Autodesk Inventor part; units mm, degrees
(part 2 of 2)
sketch "Sketch10" plane through (0, 0, 0) normal (1, 0, 0) x (0, 0, -1)
  line L0 (200.5868, 90.5719) -> (65.5868, 90.5719) projected
  arc A0 (65.5868, 90.5719) -> (50.5868, 90.5719) centre (58.0868, 90.5719) ccw projected
  line L1 (50.5868, 90.5719) -> (-146.9132, 90.5719) projected
  arc A1 (-146.9132, 90.5719) -> (-164.5909, 47.8942) centre (-146.9132, 65.5719) ccw projected
  line L2 (-164.5909, 47.8942) -> (-120.1975, 3.5008) projected
  arc A2 (-120.1975, 3.5008) -> (-113.1264, 0.5719) centre (-113.1264, 10.5719) ccw projected
  line L3 (-113.1264, 0.5719) -> (48.2351, 0.5719) projected
  arc A3 (48.2351, 0.5719) -> (67.9385, 0.5719) centre (58.0868, 2.2876) ccw projected
  line L4 (67.9385, 0.5719) -> (198.2351, 0.5719) projected
  arc A4 (198.2351, 0.5719) -> (217.9385, 0.5719) centre (208.0868, 2.2876) ccw projected
  line L5 (217.9385, 0.5719) -> (338.2351, 0.5719) projected
  arc A5 (338.2351, 0.5719) -> (357.9385, 0.5719) centre (348.0868, 2.2876) ccw projected
  line L6 (357.9385, 0.5719) -> (387.824, 0.5719) projected
  arc A6 (387.824, 0.5719) -> (392.824, 1.9116) centre (387.824, 10.5719) ccw projected
  line L7 (392.824, 1.9116) -> (465.5868, 43.9213) projected
  arc A7 (465.5868, 43.9213) -> (453.0868, 90.5719) centre (453.0868, 65.5719) ccw projected
  line L8 (453.0868, 90.5719) -> (215.5868, 90.5719) projected
  arc A8 (215.5868, 90.5719) -> (200.5868, 90.5719) centre (208.0868, 90.5719) ccw projected
  line L9 (394.4234, 30.0809) -> (384.8369, 44.4607) projected
  arc A9 (384.8369, 46.6796) -> (384.8369, 44.4607) centre (386.501, 45.5701) ccw projected
  line L10 (384.8369, 46.6796) -> (394.4264, 61.0622) projected
  arc A10 (398.0904, 59.9525) -> (394.4264, 61.0622) centre (396.0904, 59.9527) ccw projected
  line L11 (398.0904, 59.9525) -> (398.0875, 31.1901) projected
  arc A11 (394.4234, 30.0809) -> (398.0875, 31.1901) centre (396.0875, 31.1903) ccw projected
  line L12 (-95.7021, 34.3299) -> (-100.8758, 44.6775) projected
  arc A12 (-100.8758, 46.4663) -> (-100.8758, 44.6775) centre (-99.087, 45.5719) ccw projected
  line L13 (-100.8758, 46.4663) -> (-95.7021, 56.8138) projected
  arc A13 (-91.9132, 55.9194) -> (-95.7021, 56.8138) centre (-93.9132, 55.9194) ccw projected
  line L14 (-91.9132, 55.9194) -> (-91.9132, 35.2244) projected
  arc A14 (-95.7021, 34.3299) -> (-91.9132, 35.2244) centre (-93.9132, 35.2244) ccw projected
  line L15 (46.0868, 47.6815) -> (11.9586, 47.6815) projected
  arc A15 (11.0641, 51.4704) -> (11.9586, 47.6815) centre (11.9586, 49.6815) ccw projected
  line L16 (11.0641, 51.4704) -> (45.1924, 68.5345) projected
  arc A16 (48.0868, 66.7457) -> (45.1924, 68.5345) centre (46.0868, 66.7457) ccw projected
  line L17 (48.0868, 66.7457) -> (48.0868, 49.6815) projected
  arc A17 (46.0868, 47.6815) -> (48.0868, 49.6815) centre (46.0868, 49.6815) ccw projected
  line L18 (278.9812, 39.5345) -> (319.3287, 19.3608) projected
  arc A18 (318.4343, 15.5719) -> (319.3287, 19.3608) centre (318.4343, 17.5719) ccw projected
  line L19 (318.4343, 15.5719) -> (237.7393, 15.5719) projected
  arc A19 (236.8448, 19.3608) -> (237.7393, 15.5719) centre (237.7393, 17.5719) ccw projected
  line L20 (236.8448, 19.3608) -> (277.1924, 39.5345) projected
  arc A20 (278.9812, 39.5345) -> (277.1924, 39.5345) centre (278.0868, 37.7457) ccw projected
  line L21 (367.8331, 75.5719) -> (388.3444, 75.5719) projected
  arc A21 (390.0084, 72.4624) -> (388.3444, 75.5719) centre (388.3444, 73.5719) ccw projected
  line L22 (390.0084, 72.4624) -> (379.7522, 57.0798) projected
  arc A22 (376.4241, 57.0798) -> (379.7522, 57.0798) centre (378.0882, 58.1892) ccw projected
  line L23 (376.4241, 57.0798) -> (366.169, 72.4625) projected
  arc A23 (367.8331, 75.5719) -> (366.169, 72.4625) centre (367.8331, 73.5719) ccw projected
  line L24 (361.7509, 61.0619) -> (371.3389, 46.6799) projected
  arc A24 (371.3388, 44.461) -> (371.3389, 46.6799) centre (369.6748, 45.5705) ccw projected
  line L25 (371.3388, 44.461) -> (361.7508, 30.0806) projected
  arc A25 (358.0868, 31.1901) -> (361.7508, 30.0806) centre (360.0868, 31.1901) ccw projected
  line L26 (358.0868, 31.1901) -> (358.0868, 59.9525) projected
  arc A26 (361.7509, 61.0619) -> (358.0868, 59.9525) centre (360.0868, 59.9525) ccw projected
  line L27 (89.1243, 75.5719) -> (177.0493, 75.5719) projected
  arc A27 (177.8875, 71.756) -> (177.0493, 75.5719) centre (177.0493, 73.5719) ccw projected
  line L28 (177.8875, 71.756) -> (133.9249, 51.4656) projected
  arc A28 (132.2487, 51.4656) -> (133.9249, 51.4656) centre (133.0868, 53.2815) ccw projected
  line L29 (132.2487, 51.4656) -> (88.2861, 71.756) projected
  arc A29 (89.1243, 75.5719) -> (88.2861, 71.756) centre (89.1243, 73.5719) ccw projected
  line L30 (-11.0188, 39.5345) -> (29.3287, 19.3608) projected
  arc A30 (28.4343, 15.5719) -> (29.3287, 19.3608) centre (28.4343, 17.5719) ccw projected
  line L31 (28.4343, 15.5719) -> (-52.2607, 15.5719) projected
  arc A31 (-53.1552, 19.3608) -> (-52.2607, 15.5719) centre (-52.2607, 17.5719) ccw projected
  line L32 (-53.1552, 19.3608) -> (-12.8076, 39.5345) projected
  arc A32 (-11.0188, 39.5345) -> (-12.8076, 39.5345) centre (-11.9132, 37.7457) ccw projected
  line L33 (-105.1244, 30.8138) -> (-98.9506, 18.4663) projected
  arc A33 (-100.7394, 15.5719) -> (-98.9506, 18.4663) centre (-100.7394, 17.5719) ccw projected
  line L34 (-100.7394, 15.5719) -> (-113.087, 15.5719) projected
  arc A34 (-114.8758, 18.4663) -> (-113.087, 15.5719) centre (-113.087, 17.5719) ccw projected
  line L35 (-114.8758, 18.4663) -> (-108.7021, 30.8138) projected
  arc A35 (-105.1244, 30.8138) -> (-108.7021, 30.8138) centre (-106.9132, 29.9194) ccw projected
  line L36 (117.2208, 43.756) -> (70.9249, 22.3887) projected
  arc A36 (68.0868, 24.2046) -> (70.9249, 22.3887) centre (70.0868, 24.2046) ccw projected
  line L37 (68.0868, 24.2046) -> (68.0868, 66.9392) projected
  arc A37 (70.9249, 68.7551) -> (68.0868, 66.9392) centre (70.0868, 66.9392) ccw projected
  line L38 (70.9249, 68.7551) -> (117.2208, 47.3878) projected
  arc A38 (117.2208, 43.756) -> (117.2208, 47.3878) centre (116.3827, 45.5719) ccw projected
  line L39 (-118.1244, 56.8138) -> (-112.9506, 46.4663) projected
  arc A39 (-112.9506, 44.6775) -> (-112.9506, 46.4663) centre (-114.7394, 45.5719) ccw projected
  line L40 (-112.9506, 44.6775) -> (-118.1244, 34.3299) projected
  arc A40 (-121.9132, 35.2244) -> (-118.1244, 34.3299) centre (-119.9132, 35.2244) ccw projected
  line L41 (-121.9132, 35.2244) -> (-121.9132, 55.9194) projected
  arc A41 (-118.1244, 56.8138) -> (-121.9132, 55.9194) centre (-119.9132, 55.9194) ccw projected
  line L42 (-71.9132, 24.3981) -> (-71.9132, 66.7457) projected
  arc A42 (-69.0188, 68.5345) -> (-71.9132, 66.7457) centre (-69.9132, 66.7457) ccw projected
  line L43 (-69.0188, 68.5345) -> (-26.6713, 47.3608) projected
  arc A43 (-26.6713, 43.783) -> (-26.6713, 47.3608) centre (-27.5657, 45.5719) ccw projected
  line L44 (-26.6713, 43.783) -> (-69.0188, 22.6093) projected
  arc A44 (-71.9132, 24.3981) -> (-69.0188, 22.6093) centre (-69.9132, 24.3981) ccw projected
  line L45 (177.0493, 15.5719) -> (89.1243, 15.5719) projected
  arc A45 (88.2861, 19.3878) -> (89.1243, 15.5719) centre (89.1243, 17.5719) ccw projected
  line L46 (88.2861, 19.3878) -> (132.2487, 39.6782) projected
  arc A46 (133.9249, 39.6782) -> (132.2487, 39.6782) centre (133.0868, 37.8623) ccw projected
  line L47 (133.9249, 39.6782) -> (177.8875, 19.3878) projected
  arc A47 (177.0493, 15.5719) -> (177.8875, 19.3878) centre (177.0493, 17.5719) ccw projected
  line L48 (330.1924, 25.1093) -> (292.8448, 43.783) projected
  arc A48 (292.8448, 47.3608) -> (292.8448, 43.783) centre (293.7393, 45.5719) ccw projected
  line L49 (292.8448, 47.3608) -> (330.1924, 66.0345) projected
  arc A49 (333.0868, 64.2457) -> (330.1924, 66.0345) centre (331.0868, 64.2457) ccw projected
  line L50 (333.0868, 64.2457) -> (333.0868, 26.8981) projected
  arc A50 (330.1924, 25.1093) -> (333.0868, 26.8981) centre (331.0868, 26.8981) ccw projected
  line L51 (379.7517, 34.0607) -> (390.0046, 18.6813) projected
  arc A51 (388.3405, 15.5719) -> (390.0046, 18.6813) centre (388.3405, 17.5719) ccw projected
  line L52 (388.3405, 15.5719) -> (367.8335, 15.5719) projected
  arc A52 (366.1695, 18.6814) -> (367.8335, 15.5719) centre (367.8335, 17.5719) ccw projected
  line L53 (366.1695, 18.6814) -> (376.4235, 34.0608) projected
  arc A53 (379.7517, 34.0607) -> (376.4235, 34.0608) centre (378.0876, 32.9513) ccw projected
  line L54 (237.7393, 75.5719) -> (318.4343, 75.5719) projected
  arc A54 (319.3287, 71.783) -> (318.4343, 75.5719) centre (318.4343, 73.5719) ccw projected
  line L55 (319.3287, 71.783) -> (278.9812, 51.6093) projected
  arc A55 (277.1924, 51.6093) -> (278.9812, 51.6093) centre (278.0868, 53.3981) ccw projected
  line L56 (277.1924, 51.6093) -> (236.8448, 71.783) projected
  arc A56 (237.7393, 75.5719) -> (236.8448, 71.783) centre (237.7393, 73.5719) ccw projected
  line L57 (196.0868, 47.6815) -> (158.6952, 47.6815) projected
  arc A57 (157.857, 51.4975) -> (158.6952, 47.6815) centre (158.6952, 49.6815) ccw projected
  line L58 (157.857, 51.4975) -> (195.2487, 68.7551) projected
  arc A58 (198.0868, 66.9392) -> (195.2487, 68.7551) centre (196.0868, 66.9392) ccw projected
  line L59 (198.0868, 66.9392) -> (198.0868, 49.6815) projected
  arc A59 (196.0868, 47.6815) -> (198.0868, 49.6815) centre (196.0868, 49.6815) ccw projected
  line L60 (-52.2607, 75.5719) -> (28.4343, 75.5719) projected
  arc A60 (29.3287, 71.783) -> (28.4343, 75.5719) centre (28.4343, 73.5719) ccw projected
  line L61 (29.3287, 71.783) -> (-11.0188, 51.6093) projected
  arc A61 (-12.8076, 51.6093) -> (-11.0188, 51.6093) centre (-11.9132, 53.3981) ccw projected
  line L62 (-12.8076, 51.6093) -> (-53.1552, 71.783) projected
  arc A62 (-52.2607, 75.5719) -> (-53.1552, 71.783) centre (-52.2607, 73.5719) ccw projected
  line L63 (-98.9506, 72.6775) -> (-105.1244, 60.3299) projected
  arc A63 (-108.7021, 60.3299) -> (-105.1244, 60.3299) centre (-106.9132, 61.2244) ccw projected
  line L64 (-108.7021, 60.3299) -> (-114.8758, 72.6775) projected
  arc A64 (-113.087, 75.5719) -> (-114.8758, 72.6775) centre (-113.087, 73.5719) ccw projected
  line L65 (-113.087, 75.5719) -> (-100.7394, 75.5719) projected
  arc A65 (-98.9506, 72.6775) -> (-100.7394, 75.5719) centre (-100.7394, 73.5719) ccw projected
  line L66 (220.9812, 68.5345) -> (263.3287, 47.3608) projected
  arc A66 (263.3287, 43.783) -> (263.3287, 47.3608) centre (262.4343, 45.5719) ccw projected
  line L67 (263.3287, 43.783) -> (220.9812, 22.6093) projected
  arc A67 (218.0868, 24.3981) -> (220.9812, 22.6093) centre (220.0868, 24.3981) ccw projected
  line L68 (218.0868, 24.3981) -> (218.0868, 66.7457) projected
  arc A68 (220.9812, 68.5345) -> (218.0868, 66.7457) centre (220.0868, 66.7457) ccw projected
  circle A69 centre (208.0868, 2.2876) radius 2.5 projected
  circle A70 centre (348.0868, 2.2876) radius 2.5 projected
  circle A71 centre (243.0868, 8.0719) radius 2.5 projected
  circle A72 centre (183.0868, 37.6815) radius 2.5 projected
  circle A73 centre (23.0868, 37.6815) radius 2.5 projected
  circle A74 centre (-81.9132, 83.0719) radius 2.5 projected
  circle A75 centre (-122.4179, 16.3278) radius 2.5 projected
  circle A76 centre (100.0868, 83.0715) radius 2.5 projected
  circle A77 centre (260.0868, 83.0715) radius 2.5 projected
  circle A78 centre (343.0868, 37.6815) radius 2.5 projected
  circle A79 centre (348.0868, 83.0719) radius 2.5 projected
  circle A80 centre (58.0868, 2.2876) radius 2.5 projected
  circle A81 centre (-81.9132, 8.0719) radius 2.5 projected
  circle A82 centre (-146.9132, 65.5719) radius 11 projected
  line L69 (413.0868, 68.5719) -> (453.0868, 68.5719) projected
  arc A83 (453.0868, 62.5719) -> (453.0868, 68.5719) centre (453.0868, 65.5719) ccw projected
  line L70 (453.0868, 62.5719) -> (413.0868, 62.5719) projected
  arc A84 (413.0868, 68.5719) -> (413.0868, 62.5719) centre (413.0868, 65.5719) ccw projected
  line L71 (-71.9132, 24.3981) -> (-71.9132, 66.7457) projected
  line L72 (-71.9132, 24.3981) -> (-91.9132, 24.3981)
  line L73 (-91.9132, 24.3981) -> (-91.9132, 90.5719)
  line L74 (-91.9132, 90.5719) -> (-71.9132, 90.5719)
  line L75 (-71.9132, 90.5719) -> (-71.9132, 24.3981)
  line L76 (-91.9132, 90.5719) -> (-71.9132, 90.5719)
  line L77 (-71.9132, 90.5719) -> (-71.9132, -7.7124)
  line L78 (-71.9132, -7.7124) -> (-91.9132, -7.7124)
  line L79 (-91.9132, -7.7124) -> (-91.9132, 90.5719)
  line L80 (-71.9132, 90.5719) -> (-91.9132, 90.5719)
  line L81 (-91.9132, 90.5719) -> (-91.9132, 103.5219)
  line L82 (-91.9132, 103.5219) -> (-71.9132, 103.5219)
  line L83 (-71.9132, 103.5219) -> (-71.9132, 90.5719)
  point P0 (0, 0)
  point P1 (-91.9132, 0.5719)
  dimension "d165" = 20
  constraints: 24 end point, 6 parallel, 3 horizontal, 3 perpendicular, 3 point on line
  measures "d165" distance of L73.end L74.end
extrude "Extrusion4" cut sketch "Sketch10" against normal blind 10 contours L73 A13 L13 A12 L12 A14 L79 L3 A2 L2 A1 L1
sketch "Sketch11" plane through (0, 0, 0) normal (1, 0, 0) x (0, 0, -1)
  line L0 (-91.9132, 90.5719) -> (-91.9132, 0.5719) projected
  line L1 (-91.9132, 0.5719) -> (48.2351, 0.5719) projected
  arc A0 (48.2351, 0.5719) -> (67.9385, 0.5719) centre (58.0868, 2.2876) ccw projected
  line L2 (67.9385, 0.5719) -> (198.2351, 0.5719) projected
  arc A1 (198.2351, 0.5719) -> (217.9385, 0.5719) centre (208.0868, 2.2876) ccw projected
  line L3 (217.9385, 0.5719) -> (338.2351, 0.5719) projected
  arc A2 (338.2351, 0.5719) -> (357.9385, 0.5719) centre (348.0868, 2.2876) ccw projected
  line L4 (357.9385, 0.5719) -> (387.824, 0.5719) projected
  arc A3 (387.824, 0.5719) -> (392.824, 1.9116) centre (387.824, 10.5719) ccw projected
  line L5 (392.824, 1.9116) -> (465.5868, 43.9213) projected
  arc A4 (465.5868, 43.9213) -> (453.0868, 90.5719) centre (453.0868, 65.5719) ccw projected
  line L6 (453.0868, 90.5719) -> (215.5868, 90.5719) projected
  arc A5 (215.5868, 90.5719) -> (200.5868, 90.5719) centre (208.0868, 90.5719) ccw projected
  line L7 (200.5868, 90.5719) -> (65.5868, 90.5719) projected
  arc A6 (65.5868, 90.5719) -> (50.5868, 90.5719) centre (58.0868, 90.5719) ccw projected
  line L8 (50.5868, 90.5719) -> (-91.9132, 90.5719) projected
  line L9 (394.4234, 30.0809) -> (384.8369, 44.4607) projected
  arc A7 (384.8369, 46.6796) -> (384.8369, 44.4607) centre (386.501, 45.5701) ccw projected
  line L10 (384.8369, 46.6796) -> (394.4264, 61.0622) projected
  arc A8 (398.0904, 59.9525) -> (394.4264, 61.0622) centre (396.0904, 59.9527) ccw projected
  line L11 (398.0904, 59.9525) -> (398.0875, 31.1901) projected
  arc A9 (394.4234, 30.0809) -> (398.0875, 31.1901) centre (396.0875, 31.1903) ccw projected
  line L12 (46.0868, 47.6815) -> (11.9586, 47.6815) projected
  arc A10 (11.0641, 51.4704) -> (11.9586, 47.6815) centre (11.9586, 49.6815) ccw projected
  line L13 (11.0641, 51.4704) -> (45.1924, 68.5345) projected
  arc A11 (48.0868, 66.7457) -> (45.1924, 68.5345) centre (46.0868, 66.7457) ccw projected
  line L14 (48.0868, 66.7457) -> (48.0868, 49.6815) projected
  arc A12 (46.0868, 47.6815) -> (48.0868, 49.6815) centre (46.0868, 49.6815) ccw projected
  line L15 (278.9812, 39.5345) -> (319.3287, 19.3608) projected
  arc A13 (318.4343, 15.5719) -> (319.3287, 19.3608) centre (318.4343, 17.5719) ccw projected
  line L16 (318.4343, 15.5719) -> (237.7393, 15.5719) projected
  arc A14 (236.8448, 19.3608) -> (237.7393, 15.5719) centre (237.7393, 17.5719) ccw projected
  line L17 (236.8448, 19.3608) -> (277.1924, 39.5345) projected
  arc A15 (278.9812, 39.5345) -> (277.1924, 39.5345) centre (278.0868, 37.7457) ccw projected
  line L18 (367.8331, 75.5719) -> (388.3444, 75.5719) projected
  arc A16 (390.0084, 72.4624) -> (388.3444, 75.5719) centre (388.3444, 73.5719) ccw projected
  line L19 (390.0084, 72.4624) -> (379.7522, 57.0798) projected
  arc A17 (376.4241, 57.0798) -> (379.7522, 57.0798) centre (378.0882, 58.1892) ccw projected
  line L20 (376.4241, 57.0798) -> (366.169, 72.4625) projected
  arc A18 (367.8331, 75.5719) -> (366.169, 72.4625) centre (367.8331, 73.5719) ccw projected
  line L21 (361.7509, 61.0619) -> (371.3389, 46.6799) projected
  arc A19 (371.3388, 44.461) -> (371.3389, 46.6799) centre (369.6748, 45.5705) ccw projected
  line L22 (371.3388, 44.461) -> (361.7508, 30.0806) projected
  arc A20 (358.0868, 31.1901) -> (361.7508, 30.0806) centre (360.0868, 31.1901) ccw projected
  line L23 (358.0868, 31.1901) -> (358.0868, 59.9525) projected
  arc A21 (361.7509, 61.0619) -> (358.0868, 59.9525) centre (360.0868, 59.9525) ccw projected
  line L24 (89.1243, 75.5719) -> (177.0493, 75.5719) projected
  arc A22 (177.8875, 71.756) -> (177.0493, 75.5719) centre (177.0493, 73.5719) ccw projected
  line L25 (177.8875, 71.756) -> (133.9249, 51.4656) projected
  arc A23 (132.2487, 51.4656) -> (133.9249, 51.4656) centre (133.0868, 53.2815) ccw projected
  line L26 (132.2487, 51.4656) -> (88.2861, 71.756) projected
  arc A24 (89.1243, 75.5719) -> (88.2861, 71.756) centre (89.1243, 73.5719) ccw projected
  line L27 (-11.0188, 39.5345) -> (29.3287, 19.3608) projected
  arc A25 (28.4343, 15.5719) -> (29.3287, 19.3608) centre (28.4343, 17.5719) ccw projected
  line L28 (28.4343, 15.5719) -> (-52.2607, 15.5719) projected
  arc A26 (-53.1552, 19.3608) -> (-52.2607, 15.5719) centre (-52.2607, 17.5719) ccw projected
  line L29 (-53.1552, 19.3608) -> (-12.8076, 39.5345) projected
  arc A27 (-11.0188, 39.5345) -> (-12.8076, 39.5345) centre (-11.9132, 37.7457) ccw projected
  line L30 (117.2208, 43.756) -> (70.9249, 22.3887) projected
  arc A28 (68.0868, 24.2046) -> (70.9249, 22.3887) centre (70.0868, 24.2046) ccw projected
  line L31 (68.0868, 24.2046) -> (68.0868, 66.9392) projected
  arc A29 (70.9249, 68.7551) -> (68.0868, 66.9392) centre (70.0868, 66.9392) ccw projected
  line L32 (70.9249, 68.7551) -> (117.2208, 47.3878) projected
  arc A30 (117.2208, 43.756) -> (117.2208, 47.3878) centre (116.3827, 45.5719) ccw projected
  line L33 (-71.9132, 24.3981) -> (-71.9132, 66.7457) projected
  arc A31 (-69.0188, 68.5345) -> (-71.9132, 66.7457) centre (-69.9132, 66.7457) ccw projected
  line L34 (-69.0188, 68.5345) -> (-26.6713, 47.3608) projected
  arc A32 (-26.6713, 43.783) -> (-26.6713, 47.3608) centre (-27.5657, 45.5719) ccw projected
  line L35 (-26.6713, 43.783) -> (-69.0188, 22.6093) projected
  arc A33 (-71.9132, 24.3981) -> (-69.0188, 22.6093) centre (-69.9132, 24.3981) ccw projected
  line L36 (177.0493, 15.5719) -> (89.1243, 15.5719) projected
  arc A34 (88.2861, 19.3878) -> (89.1243, 15.5719) centre (89.1243, 17.5719) ccw projected
  line L37 (88.2861, 19.3878) -> (132.2487, 39.6782) projected
  arc A35 (133.9249, 39.6782) -> (132.2487, 39.6782) centre (133.0868, 37.8623) ccw projected
  line L38 (133.9249, 39.6782) -> (177.8875, 19.3878) projected
  arc A36 (177.0493, 15.5719) -> (177.8875, 19.3878) centre (177.0493, 17.5719) ccw projected
  line L39 (330.1924, 25.1093) -> (292.8448, 43.783) projected
  arc A37 (292.8448, 47.3608) -> (292.8448, 43.783) centre (293.7393, 45.5719) ccw projected
  line L40 (292.8448, 47.3608) -> (330.1924, 66.0345) projected
  arc A38 (333.0868, 64.2457) -> (330.1924, 66.0345) centre (331.0868, 64.2457) ccw projected
  line L41 (333.0868, 64.2457) -> (333.0868, 26.8981) projected
  arc A39 (330.1924, 25.1093) -> (333.0868, 26.8981) centre (331.0868, 26.8981) ccw projected
  line L42 (379.7517, 34.0607) -> (390.0046, 18.6813) projected
  arc A40 (388.3405, 15.5719) -> (390.0046, 18.6813) centre (388.3405, 17.5719) ccw projected
  line L43 (388.3405, 15.5719) -> (367.8335, 15.5719) projected
  arc A41 (366.1695, 18.6814) -> (367.8335, 15.5719) centre (367.8335, 17.5719) ccw projected
  line L44 (366.1695, 18.6814) -> (376.4235, 34.0608) projected
  arc A42 (379.7517, 34.0607) -> (376.4235, 34.0608) centre (378.0876, 32.9513) ccw projected
  line L45 (237.7393, 75.5719) -> (318.4343, 75.5719) projected
  arc A43 (319.3287, 71.783) -> (318.4343, 75.5719) centre (318.4343, 73.5719) ccw projected
  line L46 (319.3287, 71.783) -> (278.9812, 51.6093) projected
  arc A44 (277.1924, 51.6093) -> (278.9812, 51.6093) centre (278.0868, 53.3981) ccw projected
  line L47 (277.1924, 51.6093) -> (236.8448, 71.783) projected
  arc A45 (237.7393, 75.5719) -> (236.8448, 71.783) centre (237.7393, 73.5719) ccw projected
  line L48 (196.0868, 47.6815) -> (158.6952, 47.6815) projected
  arc A46 (157.857, 51.4975) -> (158.6952, 47.6815) centre (158.6952, 49.6815) ccw projected
  line L49 (157.857, 51.4975) -> (195.2487, 68.7551) projected
  arc A47 (198.0868, 66.9392) -> (195.2487, 68.7551) centre (196.0868, 66.9392) ccw projected
  line L50 (198.0868, 66.9392) -> (198.0868, 49.6815) projected
  arc A48 (196.0868, 47.6815) -> (198.0868, 49.6815) centre (196.0868, 49.6815) ccw projected
  line L51 (-52.2607, 75.5719) -> (28.4343, 75.5719) projected
  arc A49 (29.3287, 71.783) -> (28.4343, 75.5719) centre (28.4343, 73.5719) ccw projected
  line L52 (29.3287, 71.783) -> (-11.0188, 51.6093) projected
  arc A50 (-12.8076, 51.6093) -> (-11.0188, 51.6093) centre (-11.9132, 53.3981) ccw projected
  line L53 (-12.8076, 51.6093) -> (-53.1552, 71.783) projected
  arc A51 (-52.2607, 75.5719) -> (-53.1552, 71.783) centre (-52.2607, 73.5719) ccw projected
  line L54 (220.9812, 68.5345) -> (263.3287, 47.3608) projected
  arc A52 (263.3287, 43.783) -> (263.3287, 47.3608) centre (262.4343, 45.5719) ccw projected
  line L55 (263.3287, 43.783) -> (220.9812, 22.6093) projected
  arc A53 (218.0868, 24.3981) -> (220.9812, 22.6093) centre (220.0868, 24.3981) ccw projected
  line L56 (218.0868, 24.3981) -> (218.0868, 66.7457) projected
  arc A54 (220.9812, 68.5345) -> (218.0868, 66.7457) centre (220.0868, 66.7457) ccw projected
  circle A55 centre (208.0868, 2.2876) radius 2.5 projected
  circle A56 centre (348.0868, 2.2876) radius 2.5 projected
  circle A57 centre (243.0868, 8.0719) radius 2.5 projected
  circle A58 centre (183.0868, 37.6815) radius 2.5 projected
  circle A59 centre (23.0868, 37.6815) radius 2.5 projected
  circle A60 centre (-81.9132, 83.0719) radius 2.5 projected
  circle A61 centre (100.0868, 83.0715) radius 2.5 projected
  circle A62 centre (260.0868, 83.0715) radius 2.5 projected
  circle A63 centre (343.0868, 37.6815) radius 2.5 projected
  circle A64 centre (348.0868, 83.0719) radius 2.5 projected
  circle A65 centre (58.0868, 2.2876) radius 2.5 projected
  circle A66 centre (-81.9132, 8.0719) radius 2.5 projected
  line L57 (413.0868, 68.5719) -> (453.0868, 68.5719) projected
  arc A67 (453.0868, 62.5719) -> (453.0868, 68.5719) centre (453.0868, 65.5719) ccw projected
  line L58 (453.0868, 62.5719) -> (413.0868, 62.5719) projected
  arc A68 (413.0868, 68.5719) -> (413.0868, 62.5719) centre (413.0868, 65.5719) ccw projected
  point P0 (0, 0)
equation "\"d28\" = 0.5 * d27"
equation "\"d30\" = d29"
equation "\"d33\" = 0.5 * d32"
equation "\"d62\" = d61"
body "Solid1"
